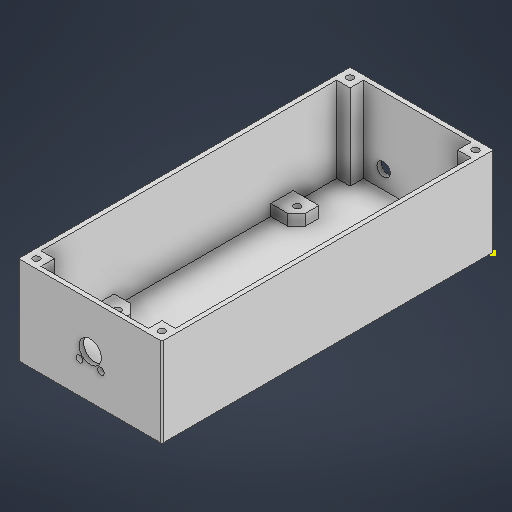
# Autodesk Inventor part: kotelo
Saved by Autodesk Inventor 2026 (Build 300175000, 175)
## iProperties
Created: 2026-01-14
Part Number: kotelo
Material: Generic
Document SubType Name: Modeling
Designer: toni.hatala
Density: 1 g/cm^3
Appearance: Default
Author: toni.hatala
Autodesk Inventor part; units mm, degrees
ref_plane "YZ Plane" through (0, 0, 0) normal (1, 0, 0) x (0, 1, 0)
ref_plane "XZ Plane" through (0, 0, 0) normal (0, 1, 0) x (-1, 0, 0)
ref_plane "XY Plane" through (0, 0, 0) normal (0, 0, 1) x (1, 0, 0)
sketch "Sketch1" plane through (0, 0, 0) normal (0, 1, 0) x (-1, 0, 0)
  line L0 (0, 0) -> (64, 0)
  line L1 (64, 0) -> (64, -148)
  line L2 (64, -148) -> (0, -148)
  line L3 (0, -148) -> (0, 0)
  dimension "d0" = 64
  dimension "d1" = 148
  constraints: 8 end point, 2 parallel, 1 horizontal, 1 perpendicular
  measures "d0" distance of L1.end L2.end
  measures "d1" distance of L0.end L1.end
extrude "Extrusion1" add sketch "Sketch1" along normal blind 40
sketch "Sketch2" plane through (0, 40, 0) normal (0, 1, 0) x (1, 0, 0)
  line L0 (-2, 2) -> (-62, 2)
  line L1 (-62, 2) -> (-62, 146)
  line L2 (-62, 146) -> (-2, 146)
  line L3 (-2, 146) -> (-2, 2)
  line L4 (-64, 148) -> (-64, 0) projected
  line L5 (0, 148) -> (-64, 148) projected
  point P0 (0, 0)
  dimension "d4" = 60
  dimension "d5" = 144
  dimension "d6" = 2
  dimension "d7" = 2
  constraints: 8 end point, 2 parallel, 1 horizontal, 1 perpendicular
  measures "d4" distance of L1.end L2.end
  measures "d5" distance of L0.end L1.end
  measures "d6" distance between parallel lines of L4 L1
  measures "d7" distance between parallel lines of L5 L2
extrude "Extrusion2" cut sketch "Sketch2" against normal blind 38
sketch "Sketch3" plane through (0, 2, 0) normal (0, 1, 0) x (1, 0, 0)
  line L0 (-2, 2) -> (-62, 2) projected
  line L1 (-62, 2) -> (-56, 2)
  line L2 (-56, 2) -> (-56, 8)
  line L3 (-56, 8) -> (-62, 8)
  line L4 (-62, 8) -> (-62, 2)
  line L5 (-62, 146) -> (-2, 146) projected
  line L6 (-62, 146) -> (-56, 146)
  line L7 (-56, 146) -> (-56, 140)
  line L8 (-56, 140) -> (-62, 140)
  line L9 (-62, 140) -> (-62, 146)
  line L10 (-2, 146) -> (-2, 2) projected
  line L11 (-2, 146) -> (-8, 146)
  line L12 (-8, 146) -> (-8, 140)
  line L13 (-8, 140) -> (-2, 140)
  line L14 (-2, 140) -> (-2, 146)
  line L15 (-2, 2) -> (-8, 2)
  line L16 (-8, 2) -> (-8, 8)
  line L17 (-8, 8) -> (-2, 8)
  line L18 (-2, 8) -> (-2, 2)
  point P0 (0, 0)
  point P1 (-2, 140)
  point P2 (-56, 2)
  point P3 (-2, 0)
  dimension "d10" = 6
  dimension "d11" = 6
  dimension "d12" = 6
  dimension "d13" = 6
  dimension "d14" = 6
  dimension "d15" = 6
  dimension "d16" = 6
  constraints: 32 end point, 8 parallel, 4 horizontal, 4 perpendicular, 1 point on line
  measures "d10" distance of L3.end L2.end
  measures "d11" distance of L2.end L1.end
  measures "d12" distance of L7.end L8.end
  measures "d13" distance of L6.end L7.end
  measures "d14" distance of L13.end L12.end
  measures "d15" distance of L12.end L11.end
  measures "d16" distance of L16.end L17.end
extrude "Extrusion3" add sketch "Sketch3" along normal blind 38
sketch "Sketch4" plane through (0, 2, 0) normal (0, 1, 0) x (1, 0, 0)
  line L0 (-59.575, 30.7653) -> (-4.425, 30.7653)
  line L1 (-4.425, 30.7653) -> (-4.425, 119.4653)
  line L2 (-4.425, 119.4653) -> (-59.575, 119.4653)
  line L3 (-59.575, 119.4653) -> (-59.575, 30.7653)
  line L4 (-62, 8) -> (-62, 146) projected
  line L5 (-2, 140) -> (-2, 8) projected
  point P0 (0, 0)
  point P1 (-62, 140)
  point P2 (-62, 2)
  dimension "d19" = 55.15
  dimension "d20" = 88.7
  dimension "d21" = 2.425
  dimension "d59" = 2.425
  constraints: 8 end point, 2 parallel, 1 horizontal, 1 perpendicular
  measures "d19" distance of L2.end L1.end
  measures "d20" distance of L1.end L0.end
  measures "d21" distance between parallel lines of L4 L3
  measures "d59" distance between parallel lines of L5 L1
extrude "Extrusion4" add sketch "Sketch4" against normal blind 2
sketch "Sketch6" plane through (0, 2, 0) normal (0, 1, 0) x (1, 0, 0)
  line L0 (-62, 8) -> (-62, 140) projected
  line L1 (-62, 30.6585) -> (-50.5, 30.6585)
  line L2 (-50.5, 30.6585) -> (-50.5, 40.6585)
  line L3 (-50.5, 40.6585) -> (-62, 40.6585)
  line L4 (-62, 40.6585) -> (-62, 30.6585)
  line L5 (-62, 120.5873) -> (-50.5, 120.5873)
  line L6 (-50.5, 120.5873) -> (-50.5, 110.5873)
  line L7 (-50.5, 110.5873) -> (-62, 110.5873)
  line L8 (-62, 110.5873) -> (-62, 120.5873)
  line L9 (-2, 140) -> (-2, 8) projected
  line L10 (-2, 120.5873) -> (-13.5, 120.5873)
  line L11 (-13.5, 120.5873) -> (-13.5, 110.5873)
  line L12 (-13.5, 110.5873) -> (-2, 110.5873)
  line L13 (-2, 110.5873) -> (-2, 120.5873)
  line L14 (-2, 30.6585) -> (-13.5, 30.6585)
  line L15 (-13.5, 30.6585) -> (-13.5, 40.6585)
  line L16 (-13.5, 40.6585) -> (-2, 40.6585)
  line L17 (-2, 40.6585) -> (-2, 30.6585)
  point P0 (0, 0)
  point P1 (-2, 8)
  point P2 (-2, 40.6585)
  point P3 (-2, 110.5873)
  point P4 (-62, 110.5873)
  point P5 (-61, 3)
  point P6 (-61, 147)
  point P7 (-3, 147)
  point P8 (-3, 3)
  dimension "d31" = 11.5
  dimension "d32" = 10
  dimension "d33" = 11.5
  dimension "d34" = 10
  dimension "d35" = 11.5
  dimension "d36" = 10
  dimension "d37" = 11.5
  dimension "d38" = 10
  constraints: 32 end point, 8 parallel, 4 horizontal, 4 perpendicular, 3 point on line, 5 other
  measures "d31" distance of L3.end L2.end
  measures "d32" distance of L2.end L1.end
  measures "d33" distance of L6.end L7.end
  measures "d34" distance of L5.end L6.end
  measures "d35" distance of L12.end L11.end
  measures "d36" distance of L11.end L10.end
  measures "d37" distance of L15.end L16.end
  measures "d38" distance of L14.end L15.end
extrude "Extrusion5" add sketch "Sketch6" along normal blind 5
chamfer "Chamfer1" distance 0.5 angle 45 1 edges at (0, 0, -74)
chamfer "Chamfer2" distance 0.5 angle 45 7 edges at (-32.25, 0, 0) (-64, 0, -74) (-32.25, 0, -148) (0, 20.25, -148) (0, 20.25, 0) (-64, 20, -148) (-64, 20, 0)
chamfer "Chamfer3" distance 4 angle 45 1 edges at (-50.5, 4.5, -110.5873)
chamfer "Chamfer4" distance 4 angle 45 3 edges at (-13.5, 4.5, -110.5873) (-50.5, 4.5, -40.6585) (-13.5, 4.5, -40.6585)
sketch "Sketch7" plane through (0, 7, 0) normal (0, 1, 0) x (1, 0, 0)
  circle A0 centre (-8.175, 34.8153) radius 1.5
  circle A1 centre (-8.175, 115.4153) radius 1.5
  circle A2 centre (-55.075, 35.2653) radius 1.5
  circle A3 centre (-55.075, 115.4653) radius 1.5
  line L0 (-4.425, 30.7653) -> (-4.425, 119.4653) projected
  line L1 (-59.575, 30.7653) -> (-4.425, 30.7653) projected
  point P0 (0, 0)
  dimension "d47" = 3
  dimension "d50" = 3
  dimension "d53" = 3
  dimension "d56" = 3
  dimension "d74" = 2.25
  dimension "d75" = 2.55
  constraints: 4 centre point
  measures "d47" diameter of A0
  measures "d50" diameter of A1
  measures "d53" diameter of A2
  measures "d56" diameter of A3
  measures "d74" distance edge to line of A0 L0
  measures "d75" distance edge to line of A0 L1
extrude "Extrusion6" cut sketch "Sketch7" against normal blind 2
sketch "Sketch8" plane through (0, 40, 0) normal (0, 1, 0) x (1, 0, 0)
  circle A0 centre (-4, 4) radius 1.5
  circle A1 centre (-60, 4) radius 1.5
  circle A2 centre (-60, 144) radius 1.5
  circle A3 centre (-4, 144) radius 1.5
  line L0 (0, 0.5) -> (0, 147.5) projected
  line L1 (-0.5, 148) -> (-63.5, 148) projected
  line L2 (-63.5, 0) -> (-0.5, 0) projected
  line L3 (-64, 147.5) -> (-64, 0.5) projected
  point P0 (0, 0)
  dimension "d78" = 3
  dimension "d79" = 3
  dimension "d80" = 3
  dimension "d81" = 3
  dimension "d82" = 4
  dimension "d83" = 4
  dimension "d84" = 4
  dimension "d85" = 4
  dimension "d86" = 4
  dimension "d87" = 4
  dimension "d88" = 4
  dimension "d89" = 4
  constraints: 4 centre point
  measures "d78" diameter of A0
  measures "d79" diameter of A1
  measures "d80" diameter of A2
  measures "d81" diameter of A3
  measures "d82" distance from line of L0 A3.centre
  measures "d83" distance from line of L1 A3.centre
  measures "d84" distance from line of L2 A0.centre
  measures "d85" distance from line of L0 A0.centre
  measures "d86" distance from line of L2 A1.centre
  measures "d87" distance from line of L3 A1.centre
  measures "d88" distance from line of L1 A2.centre
  measures "d89" distance from line of L3 A2.centre
extrude "Extrusion7" cut sketch "Sketch8" against normal blind 2
sketch "Sketch9" plane through (-0.5, 0.5, -148) normal (0, 0, -1) x (-1, 0, 0)
  point P0 (-0.5, -0.5)
sketch "Sketch10" plane through (-63.5, 40, 0) normal (0, 0, 1) x (1, 0, 0)
  circle A0 centre (31.5, -20) radius 5
  circle A1 centre (36.25, -25.1417) radius 1.5
  circle A2 centre (26.75, -25.1417) radius 1.5
  line L0 (63, -39.5) -> (0, -39.5) projected
  line L1 (63.5, -39.5) -> (63.5, 0) projected
  line L2 (0, 0) -> (63, 0) projected
  point P0 (63.5, -40)
  dimension "d93" = 10
  dimension "d94" = 3
  dimension "d95" = 3
  dimension "d96" = 0.5
  dimension "d97" = 0.5
  dimension "d98" = 9.5
  dimension "d101" = 32
  dimension "d104" = 20
  constraints: 3 centre point
  measures "d93" diameter of A0
  measures "d94" diameter of A1
  measures "d95" diameter of A2
  measures "d98" distance of A2.centre A1.centre
  measures "d101" distance from line of L1 A0.centre
  measures "d104" distance from line of L2 A0.centre
extrude "Extrusion8" cut sketch "Sketch10" against normal blind 3
sketch "Sketch13" plane through (-0.5, 0.5, -148) normal (0, 0, -1) x (-1, 0, 0)
  circle A0 centre (46.5, 9.5) radius 3
  line L0 (55.5, 1.5) -> (7.5, 1.5) projected
  line L1 (55.5, 39.5) -> (55.5, 1.5) projected
  point P0 (-0.5, -0.5)
  point P1 (31.2, 1)
  point P2 (7.5, 1.5)
  dimension "d116" = 6
  dimension "d117" = 8
  dimension "d118" = 9
  constraints: 1 centre point, 1 other
  measures "d116" diameter of A0
  measures "d118" distance from line of L1 A0.centre
extrude "Extrusion11" cut sketch "Sketch13" against normal blind 3
sketch "Sketch18" plane through (0, 2, 0) normal (0, 1, 0) x (1, 0, 0)
  line L0 (-56, 146) -> (-8, 146) projected
  line L1 (-28, 146) -> (-14, 146)
  line L2 (-14, 146) -> (-14, 131)
  line L3 (-14, 131) -> (-28, 131)
  line L4 (-28, 131) -> (-28, 146)
  line L5 (-8, 146) -> (-8, 140) projected
  point P0 (0, 0)
  point P1 (-14, 146)
  dimension "d126" = 14
  dimension "d127" = 15
  dimension "d128" = 6
  constraints: 8 end point, 2 parallel, 1 horizontal, 1 perpendicular, 1 point on line
  measures "d126" distance of L2.end L3.end
  measures "d127" distance of L1.end L2.end
  measures "d128" distance between parallel lines of L5 L2
sketch "Sketch19" plane through (-0.5, 0.5, -148) normal (0, 0, -1) x (-1, 0, 0)
  line L0 (15.25, 13) -> (25.75, 13)
  line L1 (25.75, 13) -> (25.75, 6.5)
  line L2 (25.75, 6.5) -> (15.25, 6.5)
  line L3 (15.25, 6.5) -> (15.25, 13)
  line L4 (55.5, 1.5) -> (7.5, 1.5) projected
  line L5 (7.5, 1.5) -> (7.5, 39.5) projected
  point P0 (-0.5, -0.5)
  point P1 (15.25, 9.75)
  dimension "d129" = 10.5
  dimension "d130" = 6.5
  dimension "d131" = 5
  dimension "d132" = 7.75
  constraints: 8 end point, 2 parallel, 1 horizontal, 1 midpoint, 1 perpendicular
  measures "d129" distance of L1.end L2.end
  measures "d130" distance of L0.end L1.end
  measures "d131" distance between parallel lines of L4 L2
  measures "d132" distance from line of L5 point (15.25, 9.75)
extrude "Extrusion12" cut sketch "Sketch19" against normal blind 2
extrude "Extrusion13" add sketch "Sketch18" along normal blind 5
sketch "Sketch20" plane through (-26.25, 7, -148) normal (0, 1, 0) x (1, 0, 0)
  circle A0 centre (9.23, -11.5) radius 1.5
  circle A1 centre (0.73, -11.5) radius 1.5
  line L0 (-1.75, -2) -> (-1.75, -17) projected
  line L1 (-1.75, -17) -> (12.25, -17) projected
  point P0 (26.25, -148)
  dimension "d137" = 3
  dimension "d138" = 3
  dimension "d139" = 5.5
  dimension "d140" = 0.98
  dimension "d141" = 4
  dimension "d142" = 4
  constraints: 2 centre point
  measures "d137" diameter of A0
  measures "d138" diameter of A1
  measures "d140" distance edge to line of A1 L0
  measures "d141" distance edge to line of A0 L1
  measures "d142" distance edge to line of A1 L1
extrude "Extrusion14" cut sketch "Sketch20" against normal blind 2
body "Solid1"
